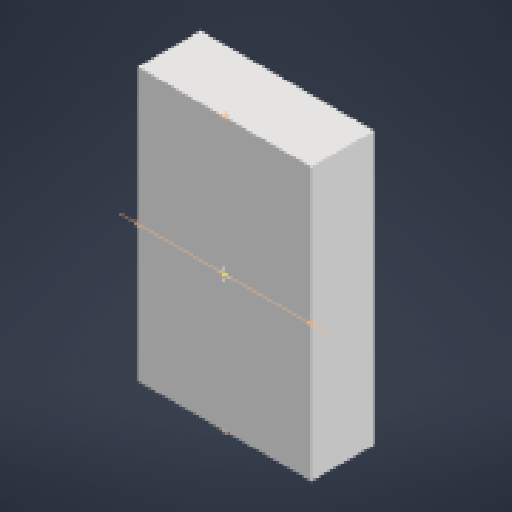
# Autodesk Inventor part: battery2
Saved by Autodesk Inventor 2026.1 (Build 301233020, 233B)
## iProperties
Created: 2026-01-13
Part Number: battery2
Material: Generic
Document SubType Name: Modeling
Designer: osama
Density: 1 g/cm^3
Appearance: Default
Author: osama
Autodesk Inventor part; units mm, degrees
ref_plane "YZ Plane" through (0, 0, 0) normal (1, 0, 0) x (0, 1, 0)
ref_plane "XZ Plane" through (0, 0, 0) normal (0, 1, 0) x (-1, 0, 0)
ref_plane "XY Plane" through (0, 0, 0) normal (0, 0, 1) x (1, 0, 0)
sketch "Sketch1" plane through (0, 0, 0) normal (0, 0, 1) x (1, 0, 0)
  line L0 (-32.5, -51) -> (32.5, -51)
  line L1 (32.5, -51) -> (32.5, 51)
  line L2 (32.5, 51) -> (-32.5, 51)
  line L3 (-32.5, 51) -> (-32.5, -51)
  line L4 (-32.5, -51) -> (32.5, 51) construction
  line L5 (32.5, -51) -> (-32.5, 51) construction
  point P0 (0, 0)
  dimension "d0" = 65
  dimension "d1" = 102
  constraints: 12 end point, 2 midpoint, 2 parallel, 1 horizontal, 1 perpendicular
  measures "d0" distance of L2.end L1.end
  measures "d1" distance of L1.end L0.end
extrude "Extrusion1" add sketch "Sketch1" along normal blind 23.5
sketch "Sketch2" plane through (0, 0, 23.5) normal (0, 0, 1) x (1, 0, 0)
  point P0 (0, 0)
  point P1 (0, 0)
  constraints: 1 coincident
body "Solid1"
